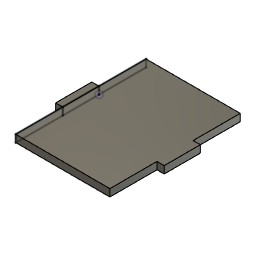
Пластина под конвейер v3 (Autodesk Fusion 360 design; units mm, degrees)
Autodesk Fusion 360 part; units mm, degrees
sketch "Sketch1" plane through (0, 0, 0) normal (1, 0, 0) x (0, 0, -1)
  line L0 (0, 0) -> (-50, 0)
  line L1 (-50, 0) -> (-50, 10)
  line L2 (-50, 10) -> (0, 10)
  line L3 (0, 10) -> (0, 0)
  line L4 (0, 0) -> (65, 0)
  line L5 (65, 0) -> (65, 10)
  line L6 (65, 10) -> (0, 10)
  line L7 (0, 10) -> (0, 0)
  line L8 (-50, 0) -> (-115, 0)
  line L9 (-115, 0) -> (-115, 10)
  line L10 (-115, 10) -> (-50, 10)
  line L11 (-50, 10) -> (-50, 0)
  dimension "d1" = 50
  dimension "d2" = 10
  dimension "d3" = 65
  dimension "d4" = 65
  dimension "d5" = 10
  dimension "d6" = 10
  constraint horizontal L0
  constraint vertical L1
  constraint horizontal L2
  constraint vertical L3
  constraint coincident L0.start L3.end
  constraint horizontal L4
  constraint vertical L5
  constraint horizontal L6
  constraint vertical L7
  constraint horizontal L8
  constraint vertical L9
  constraint horizontal L10
  constraint vertical L11
  measures "d1" distance of L0.start L0.end
  measures "d2" distance of L0.start L2.end
  measures "d3" distance of L0.start L4.end
  measures "d4" distance of L0.end L8.end
  measures "d5" distance of L8 L10
  measures "d6" distance of L4 L6
extrude "Extrude1" add sketch "Sketch1" along normal blind 130
extrude "Extrude2" add sketch "Sketch1" against normal blind 10 contours L0 L1 L2 L3 L7 L11
sketch "Sketch2" plane through (130, 0, 0) normal (1, 0, 0) x (0, 0, -1)
  line L0 (-115, 0) -> (65, 0)
  line L1 (65, 0) -> (65, 10)
  line L2 (65, 10) -> (-115, 10)
  line L3 (-115, 10) -> (-115, 0)
  line L4 (-50, 0) -> (0, 0)
  line L5 (0, 0) -> (0, 10)
  line L6 (0, 10) -> (-50, 10)
  line L7 (-50, 10) -> (-50, 0)
  constraint horizontal L4
  constraint vertical L5
  constraint horizontal L6
  constraint vertical L7
  constraint coincident L2 L5.end
  constraint coincident L0 L4.start
extrude "Extrude3" add sketch "Sketch2" along normal blind 10 contours L0 L2 L4 L5 L6 L7
